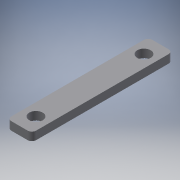
# Autodesk Inventor part: SyringeBarTail
Saved by Autodesk Inventor 2018 (Build 220112000, 112)
## iProperties
Created: 2018-10-20
Part Number: SyringeBarTail
Material: Generic
Document SubType Name: Modeling
Designer: reide
Density: 1 g/cm^3
Appearance: Default
Author: reide
Autodesk Inventor part; units mm, degrees
ref_plane "YZ Plane" through (0, 0, 0) normal (1, 0, 0) x (0, 1, 0)
ref_plane "XZ Plane" through (0, 0, 0) normal (0, 1, 0) x (-1, 0, 0)
ref_plane "XY Plane" through (0, 0, 0) normal (0, 0, 1) x (1, 0, 0)
sketch "Sketch1" plane through (0, 0, 0) normal (0, 0, 1) x (1, 0, 0)
  circle A0 centre (0, -0.002) radius 1.375 projected
  circle A1 centre (-0.0001, 26.2) radius 1.5 projected
  line L0 (0, -0.002) -> (0, -4.002)
  line L1 (0, -4.002) -> (-3, -4.002)
  line L2 (-0.0001, 26.2) -> (-3, 26.2)
  line L3 (-3, 26.2) -> (-3, 30.2)
  line L4 (-3, 30.2) -> (3, 30.2)
  line L5 (-3, -4.002) -> (3, -4.002)
  line L6 (3, -4.002) -> (3, 30.2)
  line L7 (3, 30.2) -> (-3, 30.2)
  line L8 (-3, 30.2) -> (-3, -4.002)
  circle A2 centre (0, -0.002) radius 1.625
  circle A3 centre (42.1135, 26.2) radius 1.5 projected
  circle A4 centre (-0.0001, 26.2) radius 1.5 projected
  line L9 (-6.8272, 34.4) -> (15.5728, 34.4) projected
  line L10 (-6.8272, 17) -> (-6.8272, 34.4) projected
  line L11 (48.6728, 17) -> (-6.8272, 17) projected
  line L12 (48.6728, 34.4) -> (48.6728, 17) projected
  line L13 (26.2804, 34.4) -> (48.6728, 34.4) projected
  line L14 (26.2804, 47.56) -> (26.2804, 34.4) projected
  line L15 (15.5728, 47.56) -> (26.2804, 47.56) projected
  line L16 (15.5728, 34.4) -> (15.5728, 47.56) projected
  circle A5 centre (20.9266, 44.75) radius 1.75 projected
  circle A6 centre (-0.0001, 26.2) radius 1.625
  point P0 (0, 0)
  dimension "d0" = 4
  dimension "d1" = 3
  dimension "d2" = 4
  dimension "d3" = 6
  dimension "d4" = 3.25
  dimension "d5" = 3.25
  constraints: 18 end point, 3 horizontal, 3 perpendicular, 2 centre point, 2 coincident, 2 parallel, 1 vertical
  measures "d0" distance of L0.start L0.end
  measures "d1" distance of L0.end L1.end
  measures "d2" distance of L2.end L3.end
  measures "d3" distance of L3.end L4.end
  measures "d4" diameter of A2
  measures "d5" diameter of A6
extrude "Extrusion1" add sketch "Sketch1" along normal blind 2 contours L1 L8 L11 L6 L5 | L8 L3 L4 L6 L11
fillet "Fillet1" radius 1 4 edges at (-3, -4.002, 1) (3, -4.002, 1) (3, 30.2, 1) (-3, 30.2, 1)
body "Solid1"
